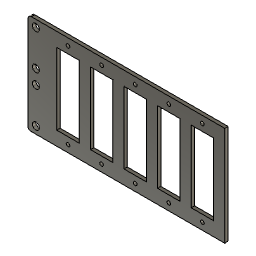
Raspberry Pi Rack Mount (Autodesk Fusion 360 design; units mm, degrees)
Autodesk Fusion 360 part; units mm, degrees
note: some values were not read from the file. Set by a fixed rule: which sketch regions a step uses.
sketch "Sketch1" plane through (0, 0, 0) normal (0, 1, 0) x (1, 0, 0)
  line L0 (0, 0) -> (15.875, 0)
  line L1 (15.875, 0) -> (15.875, -88.9)
  line L2 (15.875, -88.9) -> (0, -88.9)
  line L3 (0, -88.9) -> (0, 0)
  line L4 (0, -88.9) -> (15.875, -88.9)
  line L5 (15.875, -88.9) -> (15.875, -82.55)
  line L6 (15.875, -82.55) -> (0, -82.55)
  line L7 (0, -82.55) -> (0, -88.9)
  line L8 (0, -82.55) -> (15.875, -82.55)
  line L9 (15.875, -82.55) -> (15.875, -50.8)
  line L10 (15.875, -50.8) -> (0, -50.8)
  line L11 (0, -50.8) -> (0, -82.55)
  line L12 (0, -50.8) -> (15.875, -50.8)
  line L13 (15.875, -50.8) -> (15.875, -38.1)
  line L14 (15.875, -38.1) -> (0, -38.1)
  line L15 (0, -38.1) -> (0, -50.8)
  line L16 (0, -38.1) -> (15.875, -38.1)
  line L17 (15.875, -38.1) -> (15.875, -6.35)
  line L18 (15.875, -6.35) -> (0, -6.35)
  line L19 (0, -6.35) -> (0, -38.1)
  line L20 (15.875, -88.9) -> (18.875, -88.9)
  line L21 (18.875, -88.9) -> (18.875, 0)
  line L22 (18.875, 0) -> (15.875, 0)
  line L23 (15.875, 0) -> (15.875, -88.9)
  line L24 (15.875, -88.9) -> (7.1438, -88.9)
  line L25 (7.1438, -88.9) -> (7.1438, 0)
  line L26 (7.1438, 0) -> (15.875, 0)
  line L27 (15.875, 0) -> (15.875, -88.9)
  circle A0 centre (7.1438, -82.55) radius 3.125
  circle A1 centre (7.1438, -50.8) radius 3.125
  circle A2 centre (7.1438, -38.1) radius 3.125
  circle A3 centre (7.1438, -6.35) radius 3.125
  dimension "d1" = 15.875
  dimension "d2" = 88.9
  dimension "d3" = 6.35
  dimension "d4" = 31.75
  dimension "d5" = 12.7
  dimension "d6" = 31.75
  dimension "d7" = 3
  dimension "d8" = 8.7312
  dimension "d9" = 6.25
  dimension "d10" = 6.25
  dimension "d11" = 6.25
  dimension "d12" = 6.25
  constraint horizontal L0
  constraint vertical L1
  constraint horizontal L2
  constraint vertical L3
  constraint coincident L0.start L3.end
  constraint horizontal L4
  constraint vertical L5
  constraint horizontal L6
  constraint vertical L7
  constraint horizontal L8
  constraint vertical L9
  constraint horizontal L10
  constraint vertical L11
  constraint horizontal L12
  constraint vertical L13
  constraint horizontal L14
  constraint vertical L15
  constraint horizontal L16
  constraint vertical L17
  constraint horizontal L18
  constraint vertical L19
  constraint horizontal L20
  constraint vertical L21
  constraint horizontal L22
  constraint vertical L23
  constraint horizontal L24
  constraint vertical L25
  constraint horizontal L26
  constraint vertical L27
  constraint coincident L8 A0.centre
  constraint coincident L25 A0.centre
  constraint coincident L12 A1.centre
  constraint coincident L25 A1.centre
  constraint coincident L25 A2.centre
  constraint coincident L16 A2.centre
  constraint coincident L18 A3.centre
  constraint coincident L25 A3.centre
  measures "d1" distance of L0.start L0.end
  measures "d2" distance of L0.start L2.end
  measures "d3" distance of L2.end L6.end
  measures "d4" distance of L6.end L10.end
  measures "d5" distance of L10.end L14.end
  measures "d6" distance of L14.end L18.end
  measures "d7" distance of L1.end L20.end
  measures "d8" distance of L1.end L24.end
  measures "d9" diameter of A0
  measures "d10" diameter of A1
  measures "d11" diameter of A2
  measures "d12" diameter of A3
extrude "Extrude1" add sketch "Sketch1" along normal blind 3 contours L0 L3 L18 L25 A3 | L0 L1 L18 L23 L25 L26 L27 A3 | L3 L14 L16 L18 L19 L25 A2 A3 | L3 L10 L12 L14 L15 L16 L25 A1 A2 | L1 L14 L16 L17 L18 L23 L25 L27 A2 A3 | L3 L6 L8 L10 L11 L12 L25 A0 A1 | L1 L10 L12 L13 L14 L16 L23 L25 L27 A1 A2 | L2 L3 L4 L6 L7 L8 L25 A0 | L1 L6 L8 L9 L10 L12 L23 L25 L27 A0 A1 | L1 L2 L4 L5 L6 L8 L23 L24 L25 L27 A0
fillet "Fillet1" radius 3 1 edges at (0, 1.5, 88.9)
fillet "Fillet2" radius 3 1 edges at (0, 1.5, 0)
extrude "Extrude2" add 1 faces at (15.875, 2, 29.6333) along direction (1, 0, 0) blind 160
sketch "Sketch2" plane through (0, 0, 0) normal (0, -1, 0) x (1, 0, 0)
  circle A0 centre (7.1438, 38.1) radius 3.125
  circle A1 centre (7.1438, 50.8) radius 3.125
  circle A2 centre (7.1438, 82.55) radius 3.125
  circle A3 centre (7.1438, 6.35) radius 3.125
  arc A4 (0, 3) -> (3, 0) centre (3, 3) ccw
  line L0 (3, 0) -> (175.875, 0)
  line L1 (175.875, 0) -> (175.875, 88.9)
  line L2 (175.875, 88.9) -> (3, 88.9)
  arc A5 (3, 88.9) -> (0, 85.9) centre (3, 85.9) ccw
  line L3 (0, 85.9) -> (0, 3)
  line L4 (175.875, 88.9) -> (165.875, 88.9)
  line L5 (165.875, 88.9) -> (165.875, 0)
  line L6 (165.875, 0) -> (175.875, 0)
  line L7 (175.875, 0) -> (175.875, 88.9)
  line L8 (165.875, 88.9) -> (145.875, 88.9)
  line L9 (145.875, 88.9) -> (145.875, 0)
  line L10 (145.875, 0) -> (165.875, 0)
  line L11 (165.875, 0) -> (165.875, 88.9)
  line L12 (145.875, 88.9) -> (135.875, 88.9)
  line L13 (135.875, 88.9) -> (135.875, 0)
  line L14 (135.875, 0) -> (145.875, 0)
  line L15 (145.875, 0) -> (145.875, 88.9)
  line L16 (135.875, 88.9) -> (115.875, 88.9)
  line L17 (115.875, 88.9) -> (115.875, 0)
  line L18 (115.875, 0) -> (135.875, 0)
  line L19 (135.875, 0) -> (135.875, 88.9)
  line L20 (115.875, 88.9) -> (105.875, 88.9)
  line L21 (105.875, 88.9) -> (105.875, 0)
  line L22 (105.875, 0) -> (115.875, 0)
  line L23 (115.875, 0) -> (115.875, 88.9)
  line L24 (105.875, 88.9) -> (85.875, 88.9)
  line L25 (85.875, 88.9) -> (85.875, 0)
  line L26 (85.875, 0) -> (105.875, 0)
  line L27 (105.875, 0) -> (105.875, 88.9)
  line L28 (85.875, 88.9) -> (75.875, 88.9)
  line L29 (75.875, 88.9) -> (75.875, 0)
  line L30 (75.875, 0) -> (85.875, 0)
  line L31 (85.875, 0) -> (85.875, 88.9)
  line L32 (75.875, 88.9) -> (55.875, 88.9)
  line L33 (55.875, 88.9) -> (55.875, 0)
  line L34 (55.875, 0) -> (75.875, 0)
  line L35 (75.875, 0) -> (75.875, 88.9)
  line L36 (55.875, 88.9) -> (45.875, 88.9)
  line L37 (45.875, 88.9) -> (45.875, 0)
  line L38 (45.875, 0) -> (55.875, 0)
  line L39 (55.875, 0) -> (55.875, 88.9)
  line L40 (45.875, 88.9) -> (25.875, 88.9)
  line L41 (25.875, 88.9) -> (25.875, 0)
  line L42 (25.875, 0) -> (45.875, 0)
  line L43 (45.875, 0) -> (45.875, 88.9)
  line L44 (25.875, 88.9) -> (15.875, 88.9)
  line L45 (15.875, 88.9) -> (15.875, 0)
  line L46 (15.875, 0) -> (25.875, 0)
  line L47 (25.875, 0) -> (25.875, 88.9)
  line L48 (15.875, 0) -> (175.875, 0)
  line L49 (175.875, 0) -> (175.875, 44.45)
  line L50 (175.875, 44.45) -> (15.875, 44.45)
  line L51 (15.875, 44.45) -> (15.875, 0)
  line L52 (145.875, 44.45) -> (165.875, 44.45)
  line L53 (165.875, 44.45) -> (165.875, 76.45)
  line L54 (165.875, 76.45) -> (145.875, 76.45)
  line L55 (145.875, 76.45) -> (145.875, 44.45)
  line L56 (145.875, 44.45) -> (165.875, 44.45)
  line L57 (165.875, 44.45) -> (165.875, 12.45)
  line L58 (165.875, 12.45) -> (145.875, 12.45)
  line L59 (145.875, 12.45) -> (145.875, 44.45)
  line L60 (115.875, 44.45) -> (135.875, 44.45)
  line L61 (135.875, 44.45) -> (135.875, 76.45)
  line L62 (135.875, 76.45) -> (115.875, 76.45)
  line L63 (115.875, 76.45) -> (115.875, 44.45)
  line L64 (115.875, 44.45) -> (135.875, 44.45)
  line L65 (135.875, 44.45) -> (135.875, 12.45)
  line L66 (135.875, 12.45) -> (115.875, 12.45)
  line L67 (115.875, 12.45) -> (115.875, 44.45)
  line L68 (85.875, 44.45) -> (105.875, 44.45)
  line L69 (105.875, 44.45) -> (105.875, 76.45)
  line L70 (105.875, 76.45) -> (85.875, 76.45)
  line L71 (85.875, 76.45) -> (85.875, 44.45)
  line L72 (85.875, 44.45) -> (105.875, 44.45)
  line L73 (105.875, 44.45) -> (105.875, 12.45)
  line L74 (105.875, 12.45) -> (85.875, 12.45)
  line L75 (85.875, 12.45) -> (85.875, 44.45)
  line L76 (55.875, 44.45) -> (75.875, 44.45)
  line L77 (75.875, 44.45) -> (75.875, 76.45)
  line L78 (75.875, 76.45) -> (55.875, 76.45)
  line L79 (55.875, 76.45) -> (55.875, 44.45)
  line L80 (55.875, 44.45) -> (75.875, 44.45)
  line L81 (75.875, 44.45) -> (75.875, 12.45)
  line L82 (75.875, 12.45) -> (55.875, 12.45)
  line L83 (55.875, 12.45) -> (55.875, 44.45)
  line L84 (25.875, 44.45) -> (45.875, 44.45)
  line L85 (45.875, 44.45) -> (45.875, 76.45)
  line L86 (45.875, 76.45) -> (25.875, 76.45)
  line L87 (25.875, 76.45) -> (25.875, 44.45)
  line L88 (25.875, 44.45) -> (45.875, 44.45)
  line L89 (45.875, 44.45) -> (45.875, 12.45)
  line L90 (45.875, 12.45) -> (25.875, 12.45)
  line L91 (25.875, 12.45) -> (25.875, 44.45)
  dimension "d21" = 10
  dimension "d22" = 20
  dimension "d23" = 10
  dimension "d24" = 20
  dimension "d25" = 10
  dimension "d26" = 20
  dimension "d27" = 10
  dimension "d28" = 20
  dimension "d29" = 10
  dimension "d30" = 20
  dimension "d31" = 10
  dimension "d32" = 32
  dimension "d33" = 32
  dimension "d34" = 32
  dimension "d35" = 32
  dimension "d36" = 32
  dimension "d37" = 32
  dimension "d38" = 32
  dimension "d39" = 32
  dimension "d40" = 32
  dimension "d41" = 32
  constraint horizontal L4
  constraint vertical L5
  constraint horizontal L6
  constraint vertical L7
  constraint coincident L1.end L2.start
  constraint horizontal L8
  constraint vertical L9
  constraint horizontal L10
  constraint vertical L11
  constraint horizontal L12
  constraint vertical L13
  constraint horizontal L14
  constraint vertical L15
  constraint horizontal L16
  constraint vertical L17
  constraint horizontal L18
  constraint vertical L19
  constraint horizontal L20
  constraint vertical L21
  constraint horizontal L22
  constraint vertical L23
  constraint horizontal L24
  constraint vertical L25
  constraint horizontal L26
  constraint vertical L27
  constraint horizontal L28
  constraint vertical L29
  constraint horizontal L30
  constraint vertical L31
  constraint horizontal L32
  constraint vertical L33
  constraint horizontal L34
  constraint vertical L35
  constraint horizontal L36
  constraint vertical L37
  constraint horizontal L38
  constraint vertical L39
  constraint horizontal L40
  constraint vertical L41
  constraint horizontal L42
  constraint vertical L43
  constraint horizontal L44
  constraint vertical L45
  constraint horizontal L46
  constraint vertical L47
  constraint horizontal L48
  constraint vertical L49
  constraint horizontal L50
  constraint vertical L51
  constraint midpoint L1 L49.end
  constraint horizontal L52
  constraint vertical L53
  constraint horizontal L54
  constraint vertical L55
  constraint midpoint L15 L52.start
  constraint horizontal L56
  constraint vertical L57
  constraint horizontal L58
  constraint vertical L59
  constraint horizontal L60
  constraint vertical L61
  constraint horizontal L62
  constraint vertical L63
  constraint midpoint L23 L60.start
  constraint horizontal L64
  constraint vertical L65
  constraint horizontal L66
  constraint vertical L67
  constraint horizontal L68
  constraint vertical L69
  constraint horizontal L70
  constraint vertical L71
  constraint midpoint L25 L68.start
  constraint horizontal L72
  constraint vertical L73
  constraint horizontal L74
  constraint vertical L75
  constraint horizontal L76
  constraint vertical L77
  constraint horizontal L78
  constraint vertical L79
  constraint midpoint L39 L76.start
  constraint horizontal L80
  constraint vertical L81
  constraint horizontal L82
  constraint vertical L83
  constraint horizontal L84
  constraint vertical L85
  constraint horizontal L86
  constraint vertical L87
  constraint midpoint L47 L84.start
  constraint horizontal L88
  constraint vertical L89
  constraint horizontal L90
  constraint vertical L91
  measures "d21" distance of L1.end L4.end
  measures "d22" distance of L4.end L8.end
  measures "d23" distance of L8.end L12.end
  measures "d24" distance of L12.end L16.end
  measures "d25" distance of L16.end L20.end
  measures "d26" distance of L20.end L24.end
  measures "d27" distance of L24.end L28.end
  measures "d28" distance of L28.end L32.end
  measures "d29" distance of L32.end L36.end
  measures "d30" distance of L36.end L40.end
  measures "d31" distance of L40.end L44.end
  measures "d32" distance of L52.start L54.end
  measures "d33" distance of L52.start L58.end
  measures "d34" distance of L60.start L62.end
  measures "d35" distance of L60.start L66.end
  measures "d36" distance of L68.start L70.end
  measures "d37" distance of L68.start L74.end
  measures "d38" distance of L76.start L78.end
  measures "d39" distance of L76.start L82.end
  measures "d40" distance of L84.start L86.end
  measures "d41" distance of L84.start L90.end
extrude "Extrude3" cut sketch "Sketch2" against normal blind 3 contours L37 L41 L43 L47 L50 L84 L88 L89 L90 L91 | L37 L41 L43 L47 L50 L84 L85 L86 L87 L88 | L29 L33 L35 L39 L50 L76 L80 L81 L82 L83 | L29 L33 L35 L39 L50 L76 L77 L78 L79 L80 | L21 L25 L27 L31 L50 L68 L72 L73 L74 L75 | L21 L25 L27 L31 L50 L68 L69 L70 L71 L72 | L13 L17 L19 L23 L50 L60 L64 L65 L66 L67 | L13 L17 L19 L23 L50 L60 L61 L62 L63 L64 | L5 L9 L11 L15 L50 L52 L56 L57 L58 L59 | L5 L9 L11 L15 L50 L52 L53 L54 L55 L56
sketch "Sketch3" plane through (0, 0, 0) normal (0, -1, 0) x (1, 0, 0)
  line L0 (85.875, 76.45) -> (105.875, 76.45)
  line L1 (105.875, 76.45) -> (105.875, 12.45)
  line L2 (105.875, 12.45) -> (85.875, 12.45)
  line L3 (85.875, 12.45) -> (85.875, 76.45)
  line L4 (55.875, 76.45) -> (75.875, 76.45)
  line L5 (75.875, 76.45) -> (75.875, 12.45)
  line L6 (75.875, 12.45) -> (55.875, 12.45)
  line L7 (55.875, 12.45) -> (55.875, 76.45)
  line L8 (115.875, 76.45) -> (135.875, 76.45)
  line L9 (135.875, 76.45) -> (135.875, 12.45)
  line L10 (135.875, 12.45) -> (115.875, 12.45)
  line L11 (115.875, 12.45) -> (115.875, 76.45)
  line L12 (25.875, 76.45) -> (45.875, 76.45)
  line L13 (45.875, 76.45) -> (45.875, 12.45)
  line L14 (45.875, 12.45) -> (25.875, 12.45)
  line L15 (25.875, 12.45) -> (25.875, 76.45)
  line L16 (145.875, 76.45) -> (165.875, 76.45)
  line L17 (165.875, 76.45) -> (165.875, 12.45)
  line L18 (165.875, 12.45) -> (145.875, 12.45)
  line L19 (145.875, 12.45) -> (145.875, 76.45)
  circle A0 centre (7.1438, 38.1) radius 3.125
  circle A1 centre (7.1438, 50.8) radius 3.125
  circle A2 centre (7.1438, 82.55) radius 3.125
  circle A3 centre (7.1438, 6.35) radius 3.125
  arc A4 (0, 3) -> (3, 0) centre (3, 3) ccw
  line L20 (3, 0) -> (175.875, 0)
  line L21 (175.875, 0) -> (175.875, 88.9)
  line L22 (175.875, 88.9) -> (3, 88.9)
  arc A5 (3, 88.9) -> (0, 85.9) centre (3, 85.9) ccw
  line L23 (0, 85.9) -> (0, 3)
  line L24 (175.875, 88.9) -> (155.875, 88.9)
  line L25 (155.875, 88.9) -> (155.875, 0)
  line L26 (155.875, 0) -> (175.875, 0)
  line L27 (175.875, 0) -> (175.875, 88.9)
  line L28 (155.875, 88.9) -> (125.875, 88.9)
  line L29 (125.875, 88.9) -> (125.875, 0)
  line L30 (125.875, 0) -> (155.875, 0)
  line L31 (155.875, 0) -> (155.875, 88.9)
  line L32 (125.875, 88.9) -> (95.875, 88.9)
  line L33 (95.875, 88.9) -> (95.875, 0)
  line L34 (95.875, 0) -> (125.875, 0)
  line L35 (125.875, 0) -> (125.875, 88.9)
  line L36 (95.875, 88.9) -> (65.875, 88.9)
  line L37 (65.875, 88.9) -> (65.875, 0)
  line L38 (65.875, 0) -> (95.875, 0)
  line L39 (95.875, 0) -> (95.875, 88.9)
  line L40 (65.875, 88.9) -> (35.875, 88.9)
  line L41 (35.875, 88.9) -> (35.875, 0)
  line L42 (35.875, 0) -> (65.875, 0)
  line L43 (65.875, 0) -> (65.875, 88.9)
  line L44 (175.875, 88.9) -> (35.875, 88.9)
  line L45 (35.875, 88.9) -> (35.875, 82.675)
  line L46 (35.875, 82.675) -> (175.875, 82.675)
  line L47 (175.875, 82.675) -> (175.875, 88.9)
  line L48 (175.875, 0) -> (35.875, 0)
  line L49 (35.875, 0) -> (35.875, 6.225)
  line L50 (35.875, 6.225) -> (175.875, 6.225)
  line L51 (175.875, 6.225) -> (175.875, 0)
  circle A6 centre (35.875, 82.675) radius 1.625
  circle A7 centre (65.875, 82.675) radius 1.625
  circle A8 centre (95.875, 82.675) radius 1.625
  circle A9 centre (125.875, 82.675) radius 1.625
  circle A10 centre (155.875, 82.675) radius 1.625
  circle A11 centre (35.875, 6.225) radius 1.625
  circle A12 centre (65.875, 6.225) radius 1.625
  circle A13 centre (95.875, 6.225) radius 1.625
  circle A14 centre (125.875, 6.225) radius 1.625
  circle A15 centre (155.875, 6.225) radius 1.625
  dimension "d44" = 20
  dimension "d45" = 30
  dimension "d46" = 30
  dimension "d47" = 30
  dimension "d48" = 30
  dimension "d49" = 6.225
  dimension "d50" = 6.225
  dimension "d51" = 3.25
  dimension "d52" = 3.25
  dimension "d53" = 3.25
  dimension "d54" = 3.25
  dimension "d55" = 3.25
  dimension "d56" = 3.25
  dimension "d57" = 3.25
  dimension "d58" = 3.25
  dimension "d59" = 3.25
  dimension "d60" = 3.25
  constraint horizontal L24
  constraint vertical L25
  constraint horizontal L26
  constraint vertical L27
  constraint coincident L21.end L22.start
  constraint horizontal L28
  constraint vertical L29
  constraint horizontal L30
  constraint vertical L31
  constraint horizontal L32
  constraint vertical L33
  constraint horizontal L34
  constraint vertical L35
  constraint horizontal L36
  constraint vertical L37
  constraint horizontal L38
  constraint vertical L39
  constraint horizontal L40
  constraint vertical L41
  constraint horizontal L42
  constraint vertical L43
  constraint horizontal L44
  constraint vertical L45
  constraint horizontal L46
  constraint vertical L47
  constraint horizontal L48
  constraint vertical L49
  constraint horizontal L50
  constraint vertical L51
  constraint coincident L45.end L46.start
  constraint coincident L43 A7.centre
  constraint coincident L46 A7.centre
  constraint coincident L39 A8.centre
  constraint coincident L46 A8.centre
  constraint coincident L35 A9.centre
  constraint coincident L46 A9.centre
  constraint coincident L46 A10.centre
  constraint coincident L25 A10.centre
  constraint coincident L49.end L50.start
  constraint coincident L43 A12.centre
  constraint coincident L50 A12.centre
  constraint coincident L39 A13.centre
  constraint coincident L50 A13.centre
  constraint coincident L35 A14.centre
  constraint coincident L50 A14.centre
  constraint coincident L25 A15.centre
  constraint coincident L50 A15.centre
  measures "d44" distance of L21.end L24.end
  measures "d45" distance of L24.end L28.end
  measures "d46" distance of L28.end L32.end
  measures "d47" distance of L32.end L36.end
  measures "d48" distance of L36.end L40.end
  measures "d49" distance of L21.end L46.end
  measures "d50" distance of L20.end L50.end
  measures "d51" diameter of A6
  measures "d52" diameter of A7
  measures "d53" diameter of A8
  measures "d54" diameter of A9
  measures "d55" diameter of A10
  measures "d56" diameter of A11
  measures "d57" diameter of A12
  measures "d58" diameter of A13
  measures "d59" diameter of A14
  measures "d60" diameter of A15
extrude "Extrude4" cut sketch "Sketch3" against normal blind 3 contours L33 L39 L46 A8 | L33 L39 L46 A8 | L33 L39 L46 A8 | L33 L39 L46 A8 | L33 L39 L50 A13 | L33 L39 L50 A13 | L37 L43 L46 A7 | L37 L43 L46 A7 | L29 L35 L46 A9 | L29 L35 L46 A9 | L33 L39 L50 A13 | L33 L39 L50 A13 | L37 L43 L46 A7 | L37 L43 L46 A7 | L29 L35 L46 A9 | L29 L35 L46 A9 | L29 L35 L50 A14 | L29 L35 L50 A14 | L37 L43 L50 A12 | L37 L43 L50 A12 | L29 L35 L50 A14 | L29 L35 L50 A14 | L37 L43 L50 A12 | L37 L43 L50 A12 | L41 L46 A6 | L41 L45 L46 A6 | L25 L31 L46 A10 | L25 L31 L46 A10 | L25 L31 L46 A10 | L41 L45 A6 | L25 L31 L46 A10 | L25 L31 L50 A15 | L25 L31 L50 A15 | L41 L49 L50 A11 | L41 L50 A11 | L41 L49 A11 | L25 L31 L50 A15 | L25 L31 L50 A15
